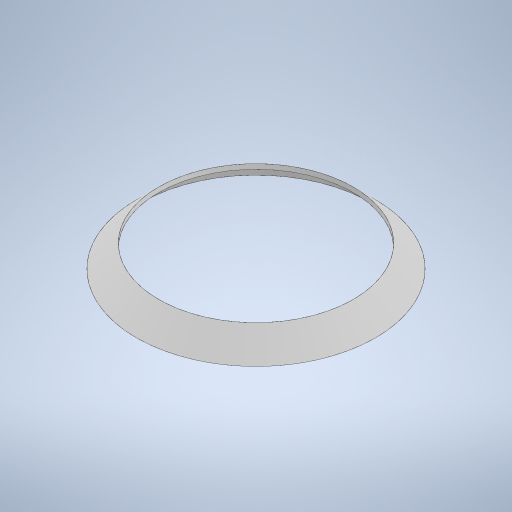
# Autodesk Inventor part: Slant
Saved by Autodesk Inventor 2024.3 (Build 283343000, 343)
## iProperties
Created: 2025-03-01
Part Number: Slant
Material: Generic
Document SubType Name: Modeling
Designer: ajclo
Density: 1 g/cm^3
Appearance: Default
Author: ajclo
Autodesk Inventor part; units mm, degrees
ref_plane "YZ Plane" through (0, 0, 0) normal (1, 0, 0) x (0, 1, 0)
ref_plane "XZ Plane" through (0, 0, 0) normal (0, 1, 0) x (-1, 0, 0)
ref_plane "XY Plane" through (0, 0, 0) normal (0, 0, 1) x (1, 0, 0)
sketch "Sketch1" plane through (0, 0, 0) normal (0, 0, 1) x (1, 0, 0)
  line L0 (70, 0) -> (57, 13)
  line L1 (57, 13) -> (57, 0)
  line L2 (57, 0) -> (70, 0)
  line L3 (67.1716, 0) -> (57, 10.1716)
  line L4 (0, 0) -> (0, 13)
  dimension "d0" = 57
  dimension "d1" = 13
  dimension "d2" = 2
  dimension "d3" = 13
  dimension "d4" = 135
  constraints: 10 end point, 2 parallel, 2 point on line, 2 vertical, 1 perpendicular
  measures "d0" distance of L4.start L1.end
  measures "d1" distance of L1.end L0.start
  measures "d2" distance between parallel lines of L0 L3
  measures "d3" distance of L0.end L1.end
  measures "d4" angle of L2 L0
revolve "Revolution1" add sketch "Sketch1" angle 360 about axis through (0, 0, 0) along (0, 1, 0) contours L2 L3 L1 L0
body "Solid1"
